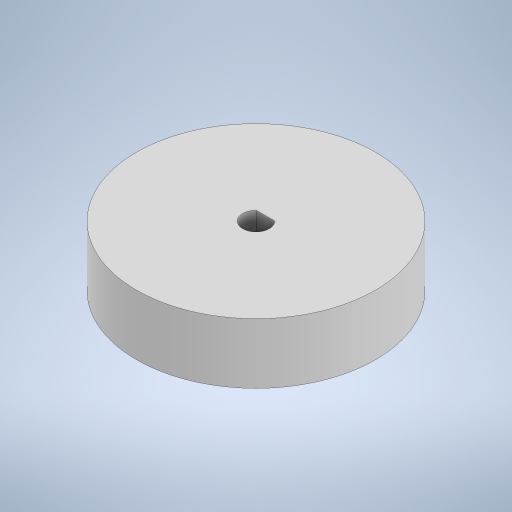
# Autodesk Inventor part: motor_gearMK2
Saved by Autodesk Inventor 2023 (Build 270158000, 158)
## iProperties
Created: 2023-03-07
Part Number: motor_gearMK2
Material: Generic
Document SubType Name: Modeling
Designer: caleb
Density: 1 g/cm^3
Appearance: Default
Author: caleb
Autodesk Inventor part; units mm, degrees
ref_plane "YZ Plane" through (0, 0, 0) normal (1, 0, 0) x (0, 1, 0)
ref_plane "XZ Plane" through (0, 0, 0) normal (0, 1, 0) x (-1, 0, 0)
ref_plane "XY Plane" through (0, 0, 0) normal (0, 0, 1) x (1, 0, 0)
sketch "Sketch1" plane through (0, 0, 0) normal (0, 1, 0) x (-1, 0, 0)
  circle A0 centre (0, 0) radius 23.75
  circle A1 centre (0, 0) radius 2.625
  line L0 (0, 2.625) -> (0, -1.875)
  line L1 (0, -1.875) -> (1.8371, -1.875)
  line L2 (0, -1.875) -> (-1.8371, -1.875)
  line L3 (27.2783, -2.4665) -> (23.263, -4.7847)
  line L4 (27.2732, 2.6035) -> (23.2311, 4.9372)
  line L5 (27.2732, 2.6035) -> (27.2783, -2.4665)
  line L6 (25.9232, 8.8418) -> (23.198, 5.0909)
  line L7 (23.8564, 13.4715) -> (25.9232, 8.8418)
  line L8 (23.8564, 13.4715) -> (19.2145, 13.9594)
  line L9 (20.0857, 18.6213) -> (19.1218, 14.0862)
  line L10 (16.3145, 22.0101) -> (20.0857, 18.6213)
  line L11 (16.3145, 22.0101) -> (11.8756, 20.5678)
  line L12 (10.7753, 25.181) -> (11.7392, 20.6459)
  line L13 (5.9518, 26.7429) -> (10.7753, 25.181)
  line L14 (5.9518, 26.7429) -> (2.4832, 23.6198)
  line L15 (-0.3983, 27.3867) -> (2.3269, 23.6357)
  line L16 (-5.4401, 26.8517) -> (-0.3983, 27.3867)
  line L17 (-5.4401, 26.8517) -> (-7.3385, 22.5878)
  line L18 (-11.503, 24.8569) -> (-7.4878, 22.5387)
  line L19 (-15.8914, 22.3175) -> (-11.503, 24.8569)
  line L20 (-15.8914, 22.3175) -> (-15.8914, 17.6501)
  line L21 (-20.6188, 18.0292) -> (-16.0078, 17.5446)
  line L22 (-23.5948, 13.9245) -> (-20.6188, 18.0292)
  line L23 (-23.5948, 13.9245) -> (-21.6964, 9.6606)
  line L24 (-26.1693, 8.0841) -> (-21.7599, 9.5168)
  line L25 (-27.2186, 3.1238) -> (-26.1693, 8.0841)
  line L26 (-27.2186, 3.1238) -> (-23.75, 0.0007)
  line L27 (-27.195, -3.2588) -> (-23.7495, -0.1565)
  line L28 (-26.1359, -8.2171) -> (-27.195, -3.2588)
  line L29 (-26.1359, -8.2171) -> (-21.697, -9.6594)
  line L30 (-23.5184, -14.0383) -> (-21.6326, -9.8027)
  line L31 (-20.5342, -18.1371) -> (-23.5184, -14.0383)
  line L32 (-20.5342, -18.1371) -> (-15.8924, -17.6492)
  line L33 (-15.7752, -22.3904) -> (-15.7752, -17.754)
  line L34 (-11.3819, -24.9211) -> (-15.7752, -22.3904)
  line L35 (-11.3819, -24.9211) -> (-7.3398, -22.5874)
  line L36 (-5.3044, -26.871) -> (-7.1902, -22.6355)
  line L37 (-0.2615, -27.396) -> (-5.3044, -26.871)
  line L38 (-0.2615, -27.396) -> (2.4819, -23.62)
  line L39 (6.0836, -26.7054) -> (2.6381, -23.603)
  line L40 (10.904, -25.1338) -> (6.0836, -26.7054)
  line L41 (10.904, -25.1338) -> (11.8744, -20.5684)
  line L42 (16.4197, -21.9221) -> (12.0103, -20.4894)
  line L43 (20.1842, -18.5258) -> (16.4197, -21.9221)
  line L44 (20.1842, -18.5258) -> (19.2138, -13.9604)
  line L45 (23.9167, -13.3484) -> (19.3057, -13.833)
  line L46 (25.9743, -8.7146) -> (23.9167, -13.3484)
  line L47 (25.9743, -8.7146) -> (23.2309, -4.9386)
  point P0 (19.2145, 13.9594)
  point P1 (23.198, 5.0909)
  point P2 (11.8756, 20.5678)
  point P3 (19.1218, 14.0862)
  point P4 (2.4832, 23.6198)
  point P5 (11.7392, 20.6459)
  point P6 (-7.3385, 22.5878)
  point P7 (2.3269, 23.6357)
  point P8 (-15.8914, 17.6501)
  point P9 (-7.4878, 22.5387)
  point P10 (-21.6964, 9.6606)
  point P11 (-16.0078, 17.5446)
  point P12 (-23.75, 0.0007)
  point P13 (-21.7599, 9.5168)
  point P14 (-21.697, -9.6594)
  point P15 (-23.7495, -0.1565)
  point P16 (-15.8924, -17.6492)
  point P17 (-21.6326, -9.8027)
  point P18 (-7.3398, -22.5874)
  point P19 (-15.7752, -17.754)
  point P20 (2.4819, -23.62)
  point P21 (-7.1902, -22.6355)
  point P22 (11.8744, -20.5684)
  point P23 (2.6381, -23.603)
  point P24 (19.2138, -13.9604)
  point P25 (12.0103, -20.4894)
  point P26 (23.2309, -4.9386)
  point P27 (19.3057, -13.833)
  dimension "d0" = 47.5
  dimension "d1" = 5.25
  dimension "d2" = 4.5
  dimension "d24" = 360
  constraints: 96 end point, 3 point on circle, 2 coincident, 1 centre point, 1 horizontal, 1 point on line, 1 vertical, 110 other
  measures "d1" diameter of A1
  measures "d2" distance of L0.start L0.end
extrude "Extrusion2" add sketch "Sketch1" along normal blind 12 contours A0 | A1 L2 L1
body "Solid2"
